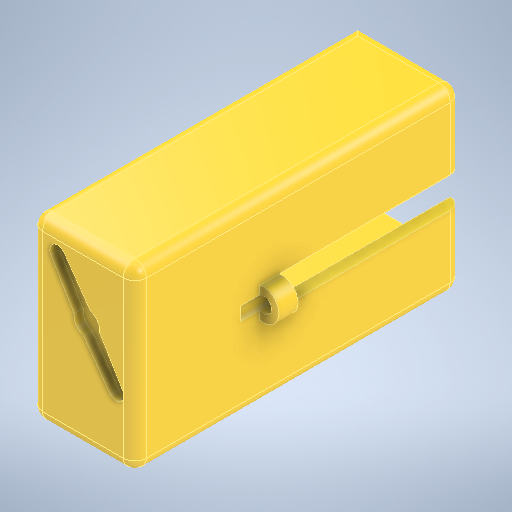
# Autodesk Inventor part: New End effector
Saved by Autodesk Inventor 2025.2 (Build 292293000, 293)
## iProperties
Created: 2025-04-03
Part Number: New End effector
Material: Generic
Document SubType Name: Modeling
Designer: abdal
Density: 1 g/cm^3
Appearance: Glossy - Gold
Author: abdal
Autodesk Inventor part; units mm, degrees
ref_plane "YZ Plane" through (0, 0, 0) normal (1, 0, 0) x (0, 1, 0)
ref_plane "XZ Plane" through (0, 0, 0) normal (0, 1, 0) x (-1, 0, 0)
sketch "Sketch1" plane through (0, 0, 0) normal (1, 0, 0) x (0, 1, 0)
  line L0 (23.289, 22.5) -> (-23.289, 22.5)
  line L1 (-23.289, 22.5) -> (-23.289, -22.5)
  line L2 (-23.289, -22.5) -> (23.289, -22.5)
  line L3 (23.289, -22.5) -> (23.289, 22.5)
  line L4 (23.289, 22.5) -> (-23.289, -22.5) construction
  line L5 (-23.289, 22.5) -> (23.289, -22.5) construction
  point P0 (0, 0)
  dimension "d0" = 45
  dimension "d1" = 46.578
  constraints: 12 end point, 2 midpoint, 2 parallel, 1 horizontal, 1 perpendicular
  measures "d0" distance of L2.end L0.start
  measures "d1" distance of L1.end L2.end
extrude "Extrusion1" add sketch "Sketch1" along normal blind 50
fillet "Fillet1" radius 0.01 2 edges at (50, 0, 22.5) (0, 0, 22.5)
sketch "Sketch2" plane through (0.01, -23.289, 22.5) normal (0, 0, 1) x (1, 0, 0)
  arc A0 (21.5019, 41.5691) -> (18.149, 39.3946) centre (19.8721, 40.41) ccw projected
  line L0 (24.1767, 29.1655) -> (18.149, 39.3946) projected
  circle A1 centre (19.7361, 40.6197) radius 0.65 projected
  circle A2 centre (20.8243, 38.9417) radius 0.65 projected
  line L1 (21.5019, 41.5691) -> (28.3834, 31.8938) projected
  circle A3 centre (21.9126, 37.2637) radius 0.65 projected
  circle A4 centre (23.0009, 35.5857) radius 0.65 projected
  circle A5 centre (24.0892, 33.9077) radius 0.65 projected
  circle A6 centre (25.1774, 32.2297) radius 0.65 projected
  circle A7 centre (29.8026, 25.0983) radius 0.65 projected
  circle A8 centre (27.49, 28.664) radius 3.325 projected
  line L2 (33.4781, 15.7589) -> (26.5966, 25.4342) projected
  arc A9 (33.4781, 15.7589) -> (36.831, 17.9334) centre (35.1079, 16.918) ccw projected
  line L3 (30.8033, 28.1625) -> (36.831, 17.9334) projected
  circle A10 centre (30.8908, 23.4203) radius 0.65 projected
  circle A11 centre (31.9791, 21.7423) radius 0.65 projected
  circle A12 centre (33.0674, 20.0643) radius 0.65 projected
  circle A13 centre (34.1557, 18.3863) radius 0.65 projected
  circle A14 centre (35.2439, 16.7083) radius 0.65 projected
  line L4 (24.1767, 29.1655) -> (24.1978, 29.1297)
  line L5 (30.8033, 28.1625) -> (30.7822, 28.1983)
  line L6 (26.5966, 25.4342) -> (26.5725, 25.4681)
  line L7 (28.3834, 31.8938) -> (28.4075, 31.8599)
  point P0 (-0.01, 23.289)
  constraints: 8 end point, 4 point on circle
extrude "Extrusion2" cut sketch "Sketch2" against normal blind 2.35 contours L1 L7 A8 L4 L0 A0 | A8 | A8 L5 L3 A9 L2 L6 | A1 | A2 | A3 | A4 | A5 | A6 | A7 | A10 | A11 | A12 | A13 | A14
sketch "Sketch3" plane through (0.01, -23.289, 22.5) normal (0, 0, 1) x (1, 0, 0)
  circle A0 centre (20.8243, 38.9417) radius 0.65 projected
  circle A1 centre (19.7361, 40.6197) radius 0.65 projected
  circle A2 centre (21.9126, 37.2637) radius 0.65 projected
  circle A3 centre (23.0009, 35.5857) radius 0.65 projected
  circle A4 centre (24.0892, 33.9077) radius 0.65 projected
  circle A5 centre (25.1774, 32.2297) radius 0.65 projected
  circle A6 centre (29.8026, 25.0983) radius 0.65 projected
  circle A7 centre (30.8908, 23.4203) radius 0.65 projected
  circle A8 centre (31.9791, 21.7423) radius 0.65 projected
  circle A9 centre (33.0674, 20.0643) radius 0.65 projected
  circle A10 centre (34.1557, 18.3863) radius 0.65 projected
  circle A11 centre (35.2439, 16.7083) radius 0.65 projected
  point P0 (-0.01, 23.289)
extrude "Extrusion3" cut sketch "Sketch3" against normal blind 10
sketch "Sketch4" plane through (50, 0, 0) normal (1, 0, 0) x (0, 0, -1)
  line L0 (30, 4) -> (30, -4) projected
  line L1 (30, -4) -> (15, -4) projected
  line L2 (15, -4) -> (15, 4) projected
  line L3 (15, 4) -> (30, 4) projected
  line L4 (62.5, 16.25) -> (-17.5, 16.25) projected
  line L5 (62.5, -16.25) -> (-17.5, -16.25) projected
  line L6 (-17.5, 16.25) -> (-17.5, -16.25) projected
  line L7 (62.5, 16.25) -> (62.5, -16.25) projected
  point P0 (0, 0)
extrude "Extrusion4" cut sketch "Sketch4" against normal through all contours L0 L1 L2 L3 | L7 L5 L6 L4
sketch "Sketch5" plane through (0, 23.289, -22.5) normal (0, 1, 0) x (1, 0, 0)
  line L0 (0, 0) -> (50, 0) projected
  line L1 (50, 0) -> (45, 0)
  line L2 (45, 0) -> (45, -48.3734)
  line L3 (45, -48.3734) -> (50, -48.3734)
  line L4 (50, -48.3734) -> (50, 0)
  point P0 (0, -22.5)
  point P1 (45, 0)
  dimension "d11" = 5
  constraints: 8 end point, 2 parallel, 1 horizontal, 1 perpendicular
  measures "d11" distance between parallel lines of L4 L2
extrude "Extrusion5" cut sketch "Sketch5" against normal through all
sketch "Sketch6" plane through (0, 23.289, 22.49) normal (0, 1, 0) x (1, 0, 0)
  line L0 (45, 4.99) -> (45, 44.99) projected
  line L1 (45, 44.99) -> (37, 44.99)
  line L2 (37, 44.99) -> (37, -0.01)
  line L3 (37, -0.01) -> (45, -0.01)
  line L4 (45, -0.01) -> (45, 44.99)
  line L5 (0.01, -0.01) -> (45, -0.01) projected
  point P0 (0, 22.49)
  point P1 (45, 9.99)
  point P2 (41, -0.01)
  point P3 (45, 9.99)
  dimension "d14" = 0
  dimension "d15" = 8
  constraints: 8 end point, 2 parallel, 1 horizontal, 1 midpoint, 1 perpendicular
  measures "d14" distance from line of L5 point (41, -0.01)
  measures "d15" distance between parallel lines of L0 L2
extrude "Extrusion6" add sketch "Sketch6" against normal up to surface (39.539 mm away)
sketch "Sketch7" plane through (0, -23.289, -22.5) normal (0, 0, -1) x (-1, 0, 0)
  line L0 (-41, 21.289) -> (-44.4641, 21.289) projected
  arc A0 (-44.4641, 21.289) -> (-41, 19.289) centre (-41, 23.289) ccw projected
  line L1 (-41, 19.289) -> (-37, 19.289) projected
  line L2 (-37, 27.289) -> (-37, 19.289) projected
  line L3 (-37, 27.289) -> (-41, 27.289) projected
  arc A1 (-41, 27.289) -> (-44.4641, 25.289) centre (-41, 23.289) ccw projected
  line L4 (-44.4641, 25.289) -> (-41, 25.289) projected
  arc A2 (-41, 21.289) -> (-41, 25.289) centre (-41, 23.289) ccw projected
  arc A3 (-44.4641, 25.289) -> (-44.4641, 21.289) centre (-41, 23.289) ccw projected
  arc A4 (-41, 25.289) -> (-41, 21.289) centre (-41, 23.289) ccw projected
  arc A5 (-41, 25.289) -> (-41, 21.289) centre (-41, 23.289) ccw projected
  line L5 (-44.4641, 25.289) -> (-41, 25.289) projected
  arc A6 (-44.4641, 25.289) -> (-44.4641, 21.289) centre (-41, 23.289) ccw projected
  line L6 (-41, 21.289) -> (-44.4641, 21.289) projected
  point P0 (0, 23.289)
sketch "Sketch8" plane through (0, 23.289, 22.49) normal (0, 1, 0) x (1, 0, 0)
  line L0 (0.01, -0.01) -> (45, -0.01) projected
  line L1 (45, -0.01) -> (40, -0.01)
  line L2 (40, -0.01) -> (40, 55.178)
  line L3 (40, 55.178) -> (45, 55.178)
  line L4 (45, 55.178) -> (45, -0.01)
  point P0 (0, 22.49)
  point P1 (40, -0.01)
  dimension "d18" = 5
  constraints: 8 end point, 2 parallel, 1 horizontal, 1 perpendicular
  measures "d18" distance between parallel lines of L4 L2
extrude "Extrusion7" cut sketch "Sketch8" against normal through all
extrude "Extrusion8" cut sketch "Sketch7" against normal blind 7.5
ref_plane "Work Plane1" through (0, 16.25, -15) normal (0, 0, -1) x (-1, 0, 0)
sketch "Sketch9" plane through (0, 16.25, -15) normal (0, 0, -1) x (-1, 0, 0)
  arc A0 (-41, -12.25) -> (-44.4641, -14.25) centre (-41, -16.25) ccw projected
  line L0 (-37, -12.25) -> (-41, -12.25) projected
  line L1 (-37, -12.25) -> (-37, -20.25) projected
  arc A1 (-41, -18.25) -> (-41, -14.25) centre (-41, -16.25) ccw projected
  arc A2 (-41, -14.25) -> (-41, -18.25) centre (-41, -16.25) ccw projected
  line L2 (-41, -18.25) -> (-44.4641, -18.25) projected
  line L3 (-44.4641, -14.25) -> (-41, -14.25) projected
  arc A3 (-44.4641, -14.25) -> (-44.4641, -18.25) centre (-41, -16.25) ccw projected
  arc A4 (-44.4641, -18.25) -> (-41, -20.25) centre (-41, -16.25) ccw projected
  line L4 (-37, -20.25) -> (-40, -20.25) projected
  line L5 (-41, -20.25) -> (-37, -20.25) projected
  line L6 (-40, -12.25) -> (-40, -20.25)
  line L7 (-40, -39.539) -> (-40, 7.039) projected
  line L8 (-39, -12.25) -> (-39, -20.25)
  point P0 (0, -16.25)
  point P1 (-39, -20.25)
  point P2 (-39, -16.25)
  constraints: 4 end point, 2 midpoint, 1 collinear, 1 point on line
extrude "Extrusion9" cut sketch "Sketch9" against normal blind 5 contours L0 L6 A1 L3 A0 | L3 A2 L2 A3 | L0 L8 A1 L6 | A1 L6 A2 | L2 A1 L6 L5 A4 | A1 L6 | L8 L4 L6 A1
extrude "Extrusion10" add sketch "Sketch9" against normal blind 5 contours L0 L6 A1 L3 A0 | L3 A2 L2 A3 | L0 L8 A1 L6 | L2 A1 L6 L5 A4 | L8 L4 L6 A1
extrude "Extrusion11" cut sketch "Sketch9" against normal blind 10 contours A1 L6 A2 | A1 L6
sketch "Sketch10" plane through (0, 23.289, 22.49) normal (0, 1, 0) x (1, 0, 0)
  line L0 (0, -0.01) -> (13, -0.01)
  line L1 (13, -0.01) -> (13, 49.0312)
  line L2 (13, 49.0312) -> (0, 49.0312)
  line L3 (0, 49.0312) -> (0, -0.01)
  line L4 (0, 44.99) -> (0, 0) projected
  line L5 (0.01, -0.01) -> (40, -0.01) projected
  point P0 (0, 22.49)
  dimension "d30" = 0
  dimension "d31" = 13
  dimension "d32" = 0
  constraints: 8 end point, 2 parallel, 1 horizontal, 1 perpendicular
  measures "d30" distance between parallel lines of L4 L3
  measures "d31" distance between parallel lines of L3 L1
  measures "d32" distance between parallel lines of L5 L0
extrude "Extrusion12" cut sketch "Sketch10" against normal through all
sketch "Sketch11" plane through (40, 4, -22.5) normal (0, 0, -1) x (-1, 0, 0)
  line L0 (27, 12.25) -> (27, 19.289) projected
  line L1 (27, 19.289) -> (0, 19.289) projected
  line L2 (0, 19.289) -> (0, 0) projected
  line L3 (0, 0) -> (3, 0) projected
  line L4 (3, 12.25) -> (3, 0) projected
  line L5 (3, 12.25) -> (27, 12.25) projected
  line L6 (27, -27.289) -> (27, -20.25) projected
  line L7 (27, -20.25) -> (3, -20.25) projected
  line L8 (3, -8) -> (3, -20.25) projected
  line L9 (3, -8) -> (0, -8) projected
  line L10 (0, -8) -> (0, -27.289) projected
  line L11 (27, -27.289) -> (0, -27.289) projected
  point P0 (40, -4)
extrude "Extrusion13" add sketch "Sketch11" along normal blind 40
fillet "Fillet2" radius 3 12 edges at (26.5, 23.289, -62.5) (40, 13.6445, -62.5) (13, 23.289, -20) (13, -23.289, -20) (26.5, -23.289, -62.5) (40, -13.6445, -62.5) (13, 0, 22.5) (40, 0, 22.5) (26.5, -23.289, 22.5) (26.5, 23.289, 22.5) (40, 23.289, -20) (40, -23.289, -20)
body "Solid1"
